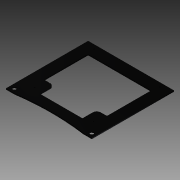
# Autodesk Inventor part: FRAME
Saved by Autodesk Inventor 2013 (Build 170138000, 138)
## iProperties
Created: 2014-03-03
Part Number: FRAME
Material: Generic
Document SubType Name: Modeling
Designer: employee
Density: 1 g/cm^3
Author: employee
Autodesk Inventor part; units mm, degrees
ref_plane "YZ Plane" through (0, 0, 0) normal (1, 0, 0) x (0, 1, 0)
ref_plane "XZ Plane" through (0, 0, 0) normal (0, 1, 0) x (-1, 0, 0)
ref_plane "XY Plane" through (0, 0, 0) normal (0, 0, 1) x (1, 0, 0)
sketch "Sketch1" plane through (0, 0, 0) normal (0, 0, 1) x (1, 0, 0)
  line L0 (262.5, -205) -> (-262.5, -205)
  line L1 (-262.5, -205) -> (-262.5, 205)
  line L2 (-262.5, 205) -> (262.5, 205)
  line L3 (262.5, 205) -> (262.5, -205)
  line L4 (-192.5, 135) -> (192.5, 135)
  line L5 (192.5, 135) -> (192.5, -135)
  line L6 (192.5, -135) -> (-192.5, -135)
  line L7 (-192.5, -135) -> (-192.5, 135)
  point P0 (0, 0)
  point P1 (-262.5, 0)
  point P2 (-192.5, 0)
  point P3 (0, 135)
  point P4 (0, 205)
  dimension "d0" = 270
  dimension "d2" = 385
  dimension "d3" = 70
  dimension "d4" = 70
  constraints: 16 end point, 4 midpoint, 4 parallel, 2 horizontal, 2 horizontal alignment, 2 perpendicular, 2 vertical alignment
  measures "d0" distance between parallel lines of L6 L4
  measures "d2" distance of L4.start L4.end
  measures "d3" distance between parallel lines of L7 L1
  measures "d4" distance between parallel lines of L2 L4
extrude "Extrusion1" add sketch "Sketch1" along normal blind 6.477
sketch "Sketch2" plane through (0, 0, 0) normal (0, 1, 0) x (-1, 0, 0)
  line L0 (192.5, 0) -> (-192.5, 0) projected
  line L1 (192.5, 0) -> (192.5, 6.477) projected
  line L2 (-192.5, 6.477) -> (192.5, 6.477) projected
  line L3 (-192.5, 0) -> (-192.5, 6.477) projected
  circle A0 centre (-157.5, 9.3054) radius 4
  circle A1 centre (157.5, 9.3054) radius 4
  line L4 (-157.5, 9.3054) -> (-154.6716, 6.477)
  line L5 (-157.5, 9.3054) -> (157.5, 9.3054)
  point P0 (0, 0)
  point P1 (0, 9.3054)
  dimension "d9" = 8
  dimension "d8" = 135
  dimension "d11" = 315
  constraints: 4 end point, 1 centre point, 1 horizontal alignment, 1 midpoint, 1 parallel, 1 point on line, 1 vertical alignment, 4 other
  measures "d8" angle of L4 L2
  measures "d11" distance of L4.start L5.end
extrude "Extrusion2" cut sketch "Sketch2" along normal mid plane 290 contours A1 L2 | L2 A1 | A0 L5 L4 L2 | L2 A0 | L4 L5 A0
sketch "Sketch3" plane through (0, 0, 6.477) normal (0, 0, 1) x (1, 0, 0)
  line L0 (-160.3284, 135) -> (-160.3284, 145) projected
  line L1 (-160.3284, 145) -> (-154.6716, 145) projected
  line L2 (-161.5, 142) -> (-153.5, 142) construction
  line L3 (-153.5, 142) -> (-153.5, 138) construction
  line L4 (-153.5, 138) -> (-161.5, 138) construction
  line L5 (-161.5, 138) -> (-161.5, 142) construction
  line L6 (-161.5, 142) -> (-163, 142)
  line L7 (-163, 142) -> (-163, 138)
  line L8 (-163, 138) -> (-161.5, 138)
  line L9 (-161.5, 138) -> (-161.5, 142)
  line L10 (-153.5, 142) -> (-152, 142)
  line L11 (-152, 142) -> (-152, 138)
  line L12 (-152, 138) -> (-153.5, 138)
  line L13 (-153.5, 138) -> (-153.5, 142)
  point P0 (0, 0)
  point P1 (-161.5, 140)
  point P2 (-160.3284, 140)
  point P3 (-157.5, 142)
  point P4 (-157.5, 145)
  dimension "d14" = 4
  dimension "d16" = 1.5
  dimension "d17" = 8
  constraints: 24 end point, 6 parallel, 4 midpoint, 3 horizontal, 3 perpendicular, 1 collinear, 1 horizontal alignment, 1 vertical alignment
  measures "d14" distance of L6.end L7.end
  measures "d16" distance of L2.start L6.end
  measures "d17" distance of L2.start L2.end
extrude "Extrusion3" cut sketch "Sketch3" against normal through all
mirror "Mirror1" about plane through (0, 0, 0) normal (0, 1, 0) of "Extrusion3"
mirror "Mirror2" about plane through (0, 0, 0) normal (1, 0, 0) of "Extrusion3", "Mirror1"
sketch "Sketch4" plane through (0, 0, 6.477) normal (0, 0, 1) x (1, 0, 0)
  line L0 (262.5, 205) -> (-262.5, 205) projected
  line L1 (-192.5, -135) -> (-192.5, 135) projected
  circle A0 centre (-201, 167.5) radius 37.5
  circle A1 centre (-201, 167.5) radius 4
  point P0 (0, 0)
  dimension "d20" = 8.5
  dimension "d21" = 8
  dimension "d22" = 75
  constraints: 2 centre point, 1 coincident, 1 tangent
  measures "d20" distance from line of A1.centre L1
  measures "d21" diameter of A1
  measures "d22" diameter of A0
extrude "Extrusion4" cut sketch "Sketch4" against normal blind 10 contours A1
mirror "Mirror3" about plane through (0, 0, 0) normal (1, 0, 0) of "Extrusion4"
sketch "Sketch5" plane through (0, 0, 6.477) normal (0, 0, 1) x (1, 0, 0)
  line L0 (154.6716, -135) -> (-154.6716, -135) projected
  line L1 (-262.5, -205) -> (262.5, -205)
  line L2 (262.5, -205) -> (262.5, -297.5)
  line L3 (262.5, -297.5) -> (-262.5, -297.5)
  line L4 (-262.5, -297.5) -> (-262.5, -205)
  point P0 (0, 0)
  dimension "d25" = 162.5
  constraints: 8 end point, 2 parallel, 1 horizontal, 1 perpendicular
  measures "d25" distance between parallel lines of L0 L3
extrude "Extrusion5" add sketch "Sketch5" against normal up to surface (6.477 mm away)
sketch "Sketch6" plane through (0, 0, 6.477) normal (0, 0, 1) x (1, 0, 0)
  line L0 (154.6716, -135) -> (-154.6716, -135) projected
  line L1 (-130, -135) -> (130, -135)
  line L2 (130, -135) -> (130, -222.5)
  line L3 (130, -222.5) -> (-130, -222.5)
  line L4 (-130, -222.5) -> (-130, -135)
  point P0 (0, 0)
  point P1 (0, -135)
  dimension "d28" = 260
  dimension "d30" = 87.5
  constraints: 8 end point, 2 midpoint, 2 parallel, 1 horizontal, 1 perpendicular, 1 point on line
  measures "d28" distance of L2.end L3.end
  measures "d30" distance of L3.end L1.start
extrude "Extrusion6" cut sketch "Sketch6" against normal through all
fillet "Fillet1" radius 25 2 edges at (-130, -135, 3.2385) (130, -135, 3.2385)
fillet "Fillet2" radius 5 4 edges at (192.5, -135, 3.2385) (192.5, 135, 3.2385) (-192.5, 135, 3.2385) (-192.5, -135, 3.2385)
sketch "Sketch7" plane through (0, 0, 6.477) normal (0, 0, 1) x (1, 0, 0)
  line L0 (-262.5, -297.5) -> (-262.5, -245.5)
  line L1 (-262.5, -245.5) -> (-210.5, -245.5)
  line L2 (-210.5, -245.5) -> (-210.5, -297.5)
  line L3 (-210.5, -297.5) -> (-262.5, -297.5)
  circle A0 centre (-236.5, -271.5) radius 11
  line L4 (-252, -256) -> (-221, -256) construction
  line L5 (-221, -256) -> (-221, -287) construction
  line L6 (-221, -287) -> (-252, -287) construction
  line L7 (-252, -287) -> (-252, -256) construction
  circle A1 centre (-221, -256) radius 1.5
  circle A2 centre (-252, -256) radius 1.5
  circle A3 centre (-252, -287) radius 1.5
  circle A4 centre (-221, -287) radius 1.5
  point P0 (0, 0)
  dimension "d35" = 52
  dimension "d36" = 22
  dimension "d37" = 31
  dimension "d38" = 3
  constraints: 16 end point, 6 coincident, 5 centre point, 3 equal radius, 2 horizontal, 18 other
  measures "d35" distance of L1.end L2.end
  measures "d36" diameter of A0
  measures "d37" distance of L4.start L4.end
  measures "d38" diameter of A2
extrude "Extrusion7" cut sketch "Sketch7" against normal through all contours A0 | A1 | A2 | A3 | A4
mirror "Mirror4" about plane through (0, 0, 0) normal (1, 0, 0) of "Extrusion7"
sketch "Sketch8" plane through (0, 0, 6.477) normal (0, 0, 1) x (1, 0, 0)
  line L0 (130, -222.5) -> (-130, -222.5) projected
  line L1 (192.5, 130) -> (192.5, -130) projected
  circle A0 centre (179, -206.5) radius 16
  circle A1 centre (179, -206.5) radius 4
  point P0 (0, 0)
  dimension "d41" = 32
  dimension "d43" = 13.5
  dimension "d45" = 8
  constraints: 2 centre point, 1 coincident, 1 tangent
  measures "d41" diameter of A0
  measures "d43" distance from line of L1 A0.centre
  measures "d45" diameter of A1
extrude "Extrusion8" cut sketch "Sketch8" against normal through all contours A1
mirror "Mirror5" about plane through (0, 0, 0) normal (1, 0, 0) of "Extrusion8"
sketch "Sketch10" plane through (0, 0, 6.477) normal (0, 0, 1) x (1, 0, 0)
  line L0 (262.5, 205) -> (-262.5, 205) projected
  line L1 (-262.5, 205) -> (-262.5, -297.5) projected
  line L2 (-262.5, -297.5) -> (262.5, -297.5) projected
  line L3 (130, -160) -> (130, -222.5) projected
  line L4 (130, -222.5) -> (-130, -222.5) projected
  line L5 (-130, -222.5) -> (-130, -160) projected
  line L6 (-80, -222.5) -> (-55, -222.5)
  line L7 (-55, -222.5) -> (-55, -216.023)
  line L8 (-55, -216.023) -> (-80, -216.023)
  line L9 (-80, -216.023) -> (-80, -222.5)
  line L10 (80, -222.5) -> (55, -222.5)
  line L11 (55, -222.5) -> (55, -216.023)
  line L12 (55, -216.023) -> (80, -216.023)
  line L13 (80, -216.023) -> (80, -222.5)
  line L14 (-262.5, -272.5) -> (-268.977, -272.5)
  line L15 (-268.977, -272.5) -> (-268.977, -247.5)
  line L16 (-268.977, -247.5) -> (-262.5, -247.5)
  line L17 (-262.5, -247.5) -> (-262.5, -272.5)
  line L18 (-262.5, -130) -> (-268.977, -130)
  line L19 (-268.977, -130) -> (-268.977, -105)
  line L20 (-268.977, -105) -> (-262.5, -105)
  line L21 (-262.5, -105) -> (-262.5, -130)
  line L22 (-262.5, 12.5) -> (-268.977, 12.5)
  line L23 (-268.977, 12.5) -> (-268.977, 37.5)
  line L24 (-268.977, 37.5) -> (-262.5, 37.5)
  line L25 (-262.5, 37.5) -> (-262.5, 12.5)
  line L26 (-262.5, 180) -> (-268.977, 180)
  line L27 (-268.977, 180) -> (-268.977, 155)
  line L28 (-268.977, 155) -> (-262.5, 155)
  line L29 (-262.5, 155) -> (-262.5, 180)
  line L30 (-268.977, -247.5) -> (-268.977, -130) construction
  line L31 (-268.977, -105) -> (-268.977, 12.5) construction
  line L32 (-268.977, 37.5) -> (-268.977, 155) construction
  point P0 (-210.5, -297.5)
  point P1 (0, 0)
  dimension "d53" = 50
  dimension "d54" = 50
  dimension "d55" = 6.477
  dimension "d56" = 25
  dimension "d57" = 25
  dimension "d58" = 6.477
  dimension "d59" = 25
  dimension "d60" = 25
  constraints: 54 end point, 14 parallel, 10 equal length, 6 horizontal, 6 perpendicular, 6 point on line, 1 collinear
  measures "d53" distance between parallel lines of L9 L5
  measures "d54" distance between parallel lines of L3 L13
  measures "d55" distance of L10.end L11.end
  measures "d56" distance of L11.end L12.end
  measures "d57" distance of L14.end L15.end
  measures "d58" distance of L14.start L14.end
  measures "d59" distance between parallel lines of L0 L26
  measures "d60" distance from line of L14.end L2
extrude "Extrusion10" add sketch "Sketch10" against normal up to surface (6.477 mm away) contours L1 L14 L15 L16 | L1 L18 L19 L20 | L1 L22 L23 L24 | L1 L28 L27 L26 | L4 L9 L8 L7
sketch "Sketch11" plane through (0, 0, 6.477) normal (0, 0, 1) x (1, 0, 0)
  line L0 (-268.977, 180) -> (-268.977, 155) projected
  line L1 (-268.977, 37.5) -> (-268.977, 12.5) projected
  line L2 (-268.977, -105) -> (-268.977, -130) projected
  line L3 (-268.977, -247.5) -> (-268.977, -272.5) projected
  line L4 (-262.5, -272.5) -> (-262.5, -297.5) projected
  line L5 (130, -222.5) -> (-55, -222.5) projected
  line L6 (-55, -216.023) -> (-80, -216.023) projected
  line L7 (-260, 169.5) -> (-258.5, 169.5)
  line L8 (-258.5, 169.5) -> (-258.5, 165.5)
  line L9 (-258.5, 165.5) -> (-260, 165.5)
  line L10 (-260, 165.5) -> (-260, 169.5)
  line L11 (-260, 27) -> (-258.5, 27)
  line L12 (-258.5, 27) -> (-258.5, 23)
  line L13 (-258.5, 23) -> (-260, 23)
  line L14 (-260, 23) -> (-260, 27)
  line L15 (-260, -115.5) -> (-258.5, -115.5)
  line L16 (-258.5, -115.5) -> (-258.5, -119.5)
  line L17 (-258.5, -119.5) -> (-260, -119.5)
  line L18 (-260, -119.5) -> (-260, -115.5)
  line L19 (-260, -258) -> (-258.5, -258)
  line L20 (-258.5, -258) -> (-258.5, -262)
  line L21 (-258.5, -262) -> (-260, -262)
  line L22 (-260, -262) -> (-260, -258)
  line L23 (-69.5, -225) -> (-65.5, -225)
  line L24 (-65.5, -225) -> (-65.5, -226.5)
  line L25 (-65.5, -226.5) -> (-69.5, -226.5)
  line L26 (-69.5, -226.5) -> (-69.5, -225)
  point P0 (0, 0)
  point P1 (-67.5, -225)
  point P2 (-67.5, -216.023)
  point P3 (-268.977, 167.5)
  point P4 (-260, 167.5)
  point P5 (-268.977, 25)
  point P6 (-260, 25)
  point P7 (-268.977, -117.5)
  point P8 (-260, -117.5)
  point P9 (-268.977, -260)
  point P10 (-260, -260)
  dimension "d63" = 2.5
  dimension "d64" = 4
  dimension "d65" = 1.5
  dimension "d66" = 2.5
  constraints: 40 end point, 10 midpoint, 10 parallel, 8 equal length, 5 horizontal, 5 perpendicular, 4 horizontal alignment, 4 vertical alignment
  measures "d63" distance between parallel lines of L5 L23
  measures "d64" distance of L21.end L19.start
  measures "d65" distance of L20.end L21.end
  measures "d66" distance between parallel lines of L22 L4
extrude "Extrusion11" cut sketch "Sketch11" against normal through all
mirror "Mirror6" about plane through (0, 0, 0) normal (1, 0, 0) of "Extrusion11", "Extrusion10"
sketch "Sketch14" plane through (0, 0, 0) normal (0, 0, -1) x (-1, 0, 0)
  line L0 (-35.5, -267.5) -> (-35.5, -287.5) projected
  line L1 (-41.977, -267.5) -> (-35.5, -267.5) projected
  line L2 (-41.977, -287.5) -> (-41.977, -267.5) projected
  line L3 (-41.977, -287.5) -> (-35.5, -287.5) projected
  line L4 (22.977, -267.5) -> (22.977, -287.5) projected
  line L5 (16.5, -267.5) -> (22.977, -267.5) projected
  line L6 (16.5, -287.5) -> (16.5, -267.5) projected
  line L7 (16.5, -287.5) -> (22.977, -287.5) projected
  line L8 (187.5, 200) -> (212.5, 200) projected
  line L9 (212.5, 200) -> (212.5, 193.523) projected
  line L10 (187.5, 193.523) -> (212.5, 193.523) projected
  line L11 (187.5, 200) -> (187.5, 193.523) projected
  line L12 (-12.5, 200) -> (12.5, 200) projected
  line L13 (12.5, 200) -> (12.5, 193.523) projected
  line L14 (-12.5, 193.523) -> (12.5, 193.523) projected
  line L15 (-12.5, 200) -> (-12.5, 193.523) projected
  line L16 (-187.5, 200) -> (-212.5, 200) projected
  line L17 (-187.5, 200) -> (-187.5, 193.523) projected
  line L18 (-187.5, 193.523) -> (-212.5, 193.523) projected
  line L19 (-212.5, 200) -> (-212.5, 193.523) projected
  line L20 (-202, 204) -> (-198, 204)
  line L21 (-198, 204) -> (-198, 202.5)
  line L22 (-198, 202.5) -> (-202, 202.5)
  line L23 (-202, 202.5) -> (-202, 204)
  line L24 (-198, 202.5) -> (-202, 202.5)
  line L25 (-202, 202.5) -> (-202, 191.023)
  line L26 (-202, 191.023) -> (-198, 191.023)
  line L27 (-198, 191.023) -> (-198, 202.5)
  line L28 (-202, 191.023) -> (-198, 191.023)
  line L29 (-198, 191.023) -> (-198, 189.523)
  line L30 (-198, 189.523) -> (-202, 189.523)
  line L31 (-202, 189.523) -> (-202, 191.023)
  line L32 (-2, 204) -> (2, 204)
  line L33 (2, 204) -> (2, 202.5)
  line L34 (2, 202.5) -> (-2, 202.5)
  line L35 (-2, 202.5) -> (-2, 204)
  line L36 (2, 202.5) -> (-2, 202.5)
  line L37 (-2, 202.5) -> (-2, 191.023)
  line L38 (-2, 191.023) -> (2, 191.023)
  line L39 (2, 191.023) -> (2, 202.5)
  line L40 (-2, 191.023) -> (2, 191.023)
  line L41 (2, 191.023) -> (2, 189.523)
  line L42 (2, 189.523) -> (-2, 189.523)
  line L43 (-2, 189.523) -> (-2, 191.023)
  line L44 (198, 204) -> (202, 204)
  line L45 (202, 204) -> (202, 202.5)
  line L46 (202, 202.5) -> (198, 202.5)
  line L47 (198, 202.5) -> (198, 204)
  line L48 (202, 202.5) -> (198, 202.5)
  line L49 (198, 202.5) -> (198, 191.023)
  line L50 (198, 191.023) -> (202, 191.023)
  line L51 (202, 191.023) -> (202, 202.5)
  line L52 (198, 191.023) -> (202, 191.023)
  line L53 (202, 191.023) -> (202, 189.523)
  line L54 (202, 189.523) -> (198, 189.523)
  line L55 (198, 189.523) -> (198, 191.023)
  line L56 (-45.977, -275.5) -> (-44.477, -275.5)
  line L57 (-44.477, -275.5) -> (-44.477, -279.5)
  line L58 (-44.477, -279.5) -> (-45.977, -279.5)
  line L59 (-45.977, -279.5) -> (-45.977, -275.5)
  line L60 (-44.477, -279.5) -> (-33, -279.5)
  line L61 (-33, -279.5) -> (-33, -275.5)
  line L62 (-33, -275.5) -> (-44.477, -275.5)
  line L63 (-44.477, -275.5) -> (-44.477, -279.5)
  line L64 (-33, -275.5) -> (-31.5, -275.5)
  line L65 (-31.5, -275.5) -> (-31.5, -279.5)
  line L66 (-31.5, -279.5) -> (-33, -279.5)
  line L67 (-33, -279.5) -> (-33, -275.5)
  line L68 (12.5, -275.5) -> (14, -275.5)
  line L69 (14, -275.5) -> (14, -279.5)
  line L70 (14, -279.5) -> (12.5, -279.5)
  line L71 (12.5, -279.5) -> (12.5, -275.5)
  line L72 (14, -279.5) -> (25.477, -279.5)
  line L73 (25.477, -279.5) -> (25.477, -275.5)
  line L74 (25.477, -275.5) -> (14, -275.5)
  line L75 (14, -275.5) -> (14, -279.5)
  line L76 (25.477, -275.5) -> (26.977, -275.5)
  line L77 (26.977, -275.5) -> (26.977, -279.5)
  line L78 (26.977, -279.5) -> (25.477, -279.5)
  line L79 (25.477, -279.5) -> (25.477, -275.5)
  point P0 (0, 0)
  point P1 (-200, 202.5)
  point P2 (-200, 200)
  point P3 (-202, 196.7615)
  point P4 (-212.5, 196.7615)
  point P5 (0, 202.5)
  point P6 (0, 200)
  point P7 (-2, 196.7615)
  point P8 (200, 202.5)
  point P9 (200, 200)
  point P10 (198, 196.7615)
  point P11 (-44.477, -277.5)
  point P12 (-41.977, -277.5)
  point P13 (-38.7385, -275.5)
  point P14 (-38.7385, -267.5)
  point P15 (14, -277.5)
  point P16 (16.5, -277.5)
  point P17 (19.7385, -275.5)
  dimension "d76" = 2.5
  dimension "d77" = 1.5
  dimension "d78" = 4
  dimension "d79" = 1.5
  dimension "d80" = 4
  dimension "d81" = 1.5
  dimension "d82" = 4
  dimension "d83" = 2.5
  dimension "d84" = 1.5
  dimension "d85" = 4
  dimension "d86" = 1.5
  dimension "d87" = 4
  constraints: 120 end point, 30 parallel, 15 equal length, 15 horizontal, 15 perpendicular, 14 midpoint, 4 vertical alignment, 3 horizontal alignment
  measures "d76" distance between parallel lines of L22 L16
  measures "d77" distance of L20.end L21.end
  measures "d78" distance of L21.end L22.end
  measures "d79" distance of L32.end L39.end
  measures "d80" distance of L39.end L34.end
  measures "d81" distance of L44.end L51.end
  measures "d82" distance of L51.end L46.end
  measures "d83" distance between parallel lines of L2 L57
  measures "d84" distance of L56.start L56.end
  measures "d85" distance of L58.end L56.start
  measures "d86" distance of L68.start L69.start
  measures "d87" distance of L70.end L68.start
extrude "Extrusion14" cut sketch "Sketch14" against normal through all contours L0 L62 L2 L1 | L0 L60 L2 L62 | L0 L3 L2 L60 | L64 L65 L66 L61 | L57 L58 L59 L56 | L4 L74 L6 L5 | L4 L72 L6 L74 | L4 L7 L6 L72 | L76 L77 L78 L73 | L69 L70 L71 L68 | L8 L49 L10 L11 | L8 L51 L10 L49 | L8 L9 L10 L51 | L47 L44 L45 L46 | L50 L53 L54 L55 | L12 L37 L14 L15 | L12 L39 L14 L37 | L12 L13 L14 L39 | L35 L32 L33 L34 | L38 L41 L42 L43 | L17 L18 L27 L16 | L27 L18 L25 L16 | L25 L18 L19 L16 | L22 L23 L20 L21 | L29 L30 L31 L26
sketch "Sketch15" plane through (0, 0, 0) normal (0, 0, -1) x (-1, 0, 0)
  line L0 (55, -222.5) -> (-55, -222.5) projected
  line L1 (-130, -222.5) -> (-130, -160) projected
  circle A0 centre (-9.5, -230) radius 5
  line L2 (-35.5, -267.5) -> (16.5, -267.5)
  point P0 (0, 0)
  point P1 (-9.5, -267.5)
  dimension "d90" = 10
  dimension "d92" = 7.5
  constraints: 2 end point, 1 centre point, 1 midpoint, 1 perpendicular, 1 vertical alignment
  measures "d90" diameter of A0
  measures "d92" distance from line of L0 A0.centre
extrude "Extrusion15" cut sketch "Sketch15" against normal through all
body "Solid1"
